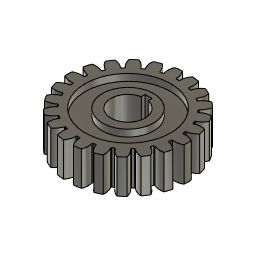
gear teeth 22 type spur gear v1 (Autodesk Fusion 360 design; units mm, degrees)
Autodesk Fusion 360 part; units mm, degrees
note: some values were not read from the file. Set by a fixed rule: which sketch regions a step uses.
sketch "Sketch1" plane through (0, 0, 0) normal (0, 0, 1) x (1, 0, 0)
  circle A0 centre (0, 0) radius 17.5
  dimension "d1" = 35
  constraint coincident A0.centre origin
  measures "d1" diameter of A0
extrude "Extrude1" add sketch "Sketch1" along normal mid plane 10
sketch "Sketch2" plane through (0, 0, 5) normal (0, 0, 1) x (-1, 0, 0)
  circle A0 centre (0, 0) radius 17.5
  circle A1 centre (0, 0) radius 5
  line L0 (0, 0) -> (0, -5) construction
  line L1 (-1, -4) -> (1, -4)
  line L2 (1, -4) -> (1, -6)
  line L3 (1, -6) -> (-1, -6)
  line L4 (-1, -6) -> (-1, -4)
  line L5 (-1, -4) -> (1, -6) construction
  line L6 (1, -4) -> (-1, -6) construction
  point P0 (0, -5)
  dimension "d4" = 10
  dimension "d5" = 2
  dimension "d6" = 2
  constraint coincident A0.centre A1.centre
  constraint coincident A1 P0
  constraint vertical L0
  constraint horizontal L1
  constraint perpendicular L1 L2
  constraint parallel L1 L3
  constraint parallel L2 L4
  constraint coincident L5 P0
  constraint coincident L6 P0
  constraint coincident P0 L0.end
  measures "d4" diameter of A1
  measures "d5" distance of L2.end L3.end
  measures "d6" distance of L1.end L2.end
extrude "Extrude2" cut sketch "Sketch2" against normal blind 10 contours A1 L1 L2 L4 | A1 L1 L2 L4 | A1 L2 L3 L4
sketch "Sketch3" plane through (0, 0, 5) normal (0, 0, 1) x (-1, 0, 0)
  line L0 (-1, -6) -> (-1, -4.899)
  arc A0 (1, -4.899) -> (-1, -4.899) centre (0, 0) ccw
  line L1 (1, -4.899) -> (1, -6)
  line L2 (1, -6) -> (-1, -6)
  circle A1 centre (0, 0) radius 17.5
  circle A2 centre (0, 0) radius 7.5
  circle A3 centre (0, 0) radius 12.5
  dimension "d9" = 15
  dimension "d10" = 25
  constraint coincident A0.centre A1.centre
  measures "d9" diameter of A2
  measures "d10" diameter of A3
extrude "Extrude3" cut sketch "Sketch3" against normal blind 2 contours A3
mirror "Mirror1" about plane through (0, 0, 0) normal (0, 0, 1) of "Extrude3"
sketch "Sketch4" plane through (0, 0, 0) normal (0, 0, 1) x (1, 0, 0)
  line L0 (0, 0) -> (0, 25) construction
  line L1 (0, 14.5) -> (0.296, 14.5)
  arc A0 (2.7, 18.5) -> (0.496, 14.6994) centre (4.896, 14.6872) ccw
  arc A1 (0.296, 14.5) -> (0.496, 14.6994) centre (0.296, 14.7) ccw
  arc A2 (-0.496, 14.6994) -> (-2.7, 18.5) centre (-4.896, 14.6872) ccw
  arc A3 (-0.496, 14.6994) -> (-0.296, 14.5) centre (-0.296, 14.7) ccw
  line L2 (0, 14.5) -> (-0.296, 14.5)
  arc A4 (2.7, 18.5) -> (-2.7, 18.5) centre (0, 11.1822) ccw
  point P0 (0.5, 14.5)
  dimension "d15" = 25
  dimension "d16" = 0.5
  dimension "d18" = 14.5
  dimension "d19" = 2.2
  dimension "d20" = 4
  dimension "d21" = 4.4
  dimension "d22" = 0.2
  dimension "d23" = 7.8
  constraint coincident L0.start origin
  constraint vertical L0
  constraint coincident L0 L1.start
  constraint horizontal L1
  constraint coincident P0 L1
  constraint coincident P0 A0
  constraint tangent A0 A1
  constraint tangent L1 A1
  constraint symmetric L0 L1.start L2.start
  constraint symmetric L0 A0.start A2.end
  constraint symmetric L0 A0 A2
  constraint symmetric L0 L1.end A3.end
  constraint symmetric L0 A0.end A2.start
  constraint symmetric L0 A1 A3
  measures "d15" distance of L0.start L0.end
  measures "d16" distance of L1.start P0
  measures "d18" vertical distance of L0.start P0
  measures "d19" horizontal distance of P0 A0.start
  measures "d20" vertical distance of P0 A0.start
  measures "d21" radius of A0
  measures "d22" radius of A1
  measures "d23" radius of A4
extrude "Extrude4" cut sketch "Sketch4" along normal mid plane 10
pattern_circular "C-Pattern1" count 22 over 360 about axis through (0, 0, 1.75) along (0, 0, 1) of "Extrude4"
